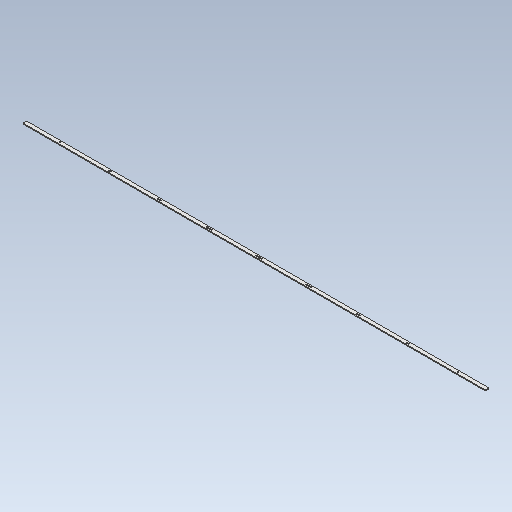
# Autodesk Inventor part: seguroAcrilico
Saved by Autodesk Inventor 2021.2 (Build 252289000, 289)
## iProperties
Created: 2026-07-28
Part Number: seguroAcrilico
Material: Generic
Document SubType Name: Sheet Metal
Designer: nelso
Density: 1 g/cm^3
Sheet Metal Rule: Default_mm
Appearance: Default
Mass: 58.4463 g
Surface Area: 475.73 cm^2
Volume: 58.4463 cm^3
Author: nelso
Autodesk Inventor part; units mm, degrees
ref_plane "YZ Plane" through (0, 0, 0) normal (1, 0, 0) x (0, 1, 0)
ref_plane "XZ Plane" through (0, 0, 0) normal (0, 1, 0) x (-1, 0, 0)
ref_plane "XY Plane" through (0, 0, 0) normal (0, 0, 1) x (1, 0, 0)
sketch "Sketch1" plane through (0, 0, 0) normal (0, 1, 0) x (-1, 0, 0)
  line L0 (-825, 6.35) -> (825, 6.35)
  line L1 (825, 6.35) -> (825, -6.35)
  line L2 (825, -6.35) -> (-825, -6.35)
  line L3 (-825, -6.35) -> (-825, 6.35)
  line L4 (-825, 6.35) -> (825, -6.35) construction
  line L5 (825, 6.35) -> (-825, -6.35) construction
  line L6 (825, 0) -> (805, 0)
  circle A0 centre (805, 0) radius 3
  circle A1 centre (630, 0) radius 3
  circle A2 centre (455, 0) radius 3
  circle A3 centre (280, 0) radius 3
  circle A4 centre (105, 0) radius 3
  circle A5 centre (-70, 0) radius 3
  circle A6 centre (-245, 0) radius 3
  circle A7 centre (-420, 0) radius 3
  circle A8 centre (-595, 0) radius 3
  circle A9 centre (-770, 0) radius 3
  point P0 (0, 0)
  dimension "d0" = 1650
  dimension "d1" = 12.7
  dimension "d3" = 20
  dimension "d4" = 6
  dimension "d7" = 175
  measures "d0" distance of L1.end L2.end
  measures "d1" distance of L0.end L1.end
  measures "d3" distance of L6.start L6.end
  measures "d4" diameter of A0
  measures "d7" distance of A0.centre A1.centre
extrude "Plate1" add sketch "Sketch1" along normal blind 3.1 contours L0 L1 L2 L3 | A0 | A1 | A2 | A3 | A4 | A5 | A6 | A7 | A8 | A9
sketch "Sketch3" plane through (0, 3.1, 0) normal (0, 1, 0) x (1, 0, 0)
  circle A0 centre (0, 0) radius 2.25
  dimension "d23" = 4.5
  constraints: 1 centre point, 1 coincident
  measures "d23" diameter of A0
extrude "Cut2" cut sketch "Sketch3" against normal blind 3.1
pattern_linear "Rectangular Pattern1" count 5 spacing 180 along (1, 0, 0) count 5 spacing 175 along (-1, 0, 0) of "Cut2"
equation "\"d24\" = Thickness"
equation "\"d2\" = Thickness"
equation "\"BendRadius\" = Thickness"
equation "\"BendReliefWidth\" = Thickness"
equation "\"BendReliefDepth\" = 0.5 * Thickness"
equation "\"CornerReliefSize\" = 4 * Thickness"
equation "\"MinimumRemnant\" = 2 * Thickness"
equation "\"TransitionRadius\" = BendRadius"
equation "\"JacobiRadiusSize\" = BendRadius"
equation "\"GapSize\" = Thickness"
equation "\"Thickness\" = 3.1"
body "Solid1"
